motor bracket_v8 (Autodesk Fusion 360 design; units mm, degrees)
Autodesk Fusion 360 part; units mm, degrees
sketch "Sketch1" plane through (0, 0, 0) normal (0, 1, 0) x (1, 0, 0) in component "Component"
  line L0 (0, 0) -> (30.5, 0)
  line L1 (0, 0) -> (0, -30.5)
  line L2 (30.5, 0) -> (30.5, -3.5)
  line L3 (0, -30.5) -> (3.5, -30.5)
  line L4 (3.5, -30.5) -> (3.5, -3.5)
  line L5 (3.5, -3.5) -> (30.5, -3.5)
  dimension "d3" = 3.5
  dimension "d4" = 3.5
  dimension "d24" = 27
  dimension "d25" = 27
  constraint coincident L0.start L1.start
  constraint horizontal L0
  constraint perpendicular L0 L1
  constraint perpendicular L0 L2
  constraint perpendicular L1 L3
  constraint perpendicular L3 L4
  constraint perpendicular L2 L5
  measures "d3" distance of L0.end L2.end
  measures "d4" distance of L1.end L3.end
  measures "d24" distance of L3.end L4.end
  measures "d25" distance of L2.end L4.end
extrude "Extrude1" add sketch "Sketch1" along normal blind 38 in component "Component"
sketch "Sketch2" plane through (3.5, 0, 0) normal (1, 0, 0) x (0, 1, 0) in component "Component"
  line L0 (0, 30.5) -> (0, 3.5)
  line L1 (0, 3.5) -> (38, 3.5)
  line L2 (38, 3.5) -> (38, 30.5)
  line L3 (38, 30.5) -> (0, 30.5)
sketch "Sketch3" plane through (0, 0, 3.5) normal (0, 0, 1) x (-1, 0, 0) in component "Component"
  line L0 (-3.5, 0) -> (-30.5, 0)
  line L1 (-30.5, 0) -> (-30.5, -38)
  line L2 (-3.5, 0) -> (-3.5, -38) construction
  line L3 (-3.5, -19) -> (-10.25, -19) construction
  line L4 (-3.5, -38) -> (-3.5, 0) construction
  line L5 (0, 0) -> (0, -38) construction
  line L6 (-10.25, -19) -> (-10.25, -28) construction
  line L7 (-10.25, -28) -> (-23.75, -28) construction
  line L8 (-10.25, -28) -> (-10.25, -32) construction
  line L9 (-10.25, -32) -> (-8.5, -32) construction
  line L10 (-10.25, -28) -> (-8.5, -28) construction
  arc A0 (-12, -32) -> (-8.5, -32) centre (-10.25, -32) ccw
  arc A1 (-8.5, -28) -> (-12, -28) centre (-10.25, -28) ccw
  line L11 (-8.5, -28) -> (-8.5, -32)
  line L12 (-12, -28) -> (-12, -32)
  line L13 (-22, -28) -> (-22, -32)
  arc A2 (-22, -28) -> (-25.5, -28) centre (-23.75, -28) ccw
  line L14 (-25.5, -28) -> (-25.5, -32)
  arc A3 (-25.5, -32) -> (-22, -32) centre (-23.75, -32) ccw
  line L15 (-8.5, -10) -> (-8.5, -6)
  arc A4 (-12, -10) -> (-8.5, -10) centre (-10.25, -10) ccw
  line L16 (-12, -10) -> (-12, -6)
  arc A5 (-8.5, -6) -> (-12, -6) centre (-10.25, -6) ccw
  line L17 (-22, -10) -> (-22, -6)
  arc A6 (-25.5, -10) -> (-22, -10) centre (-23.75, -10) ccw
  line L18 (-25.5, -10) -> (-25.5, -6)
  arc A7 (-22, -6) -> (-25.5, -6) centre (-23.75, -6) ccw
  dimension "d27" = 6.75
  dimension "d28" = 9
  dimension "d29" = 13.5
  dimension "d30" = 4
  dimension "d31" = 1.75
  dimension "d34" = -13.5
  dimension "d35" = 0
  constraint coincident L0.start L2.start
  constraint perpendicular L0 L2
  constraint midpoint L2 L3.start
  constraint perpendicular L3 L4
  constraint equal L2 L5
  constraint perpendicular L3 L6
  constraint perpendicular L6 L7
  constraint perpendicular L7 L8
  constraint perpendicular L8 L9
  constraint perpendicular L8 L10
  constraint equal L9 L10
  constraint coincident L8.end L9.start
  constraint coincident L6.end L7.start
  constraint tangent A0 L12
  constraint tangent A1 L12
  constraint symmetric L3 L9.end L15.end
  constraint symmetric L3 L10.end L15.start
  constraint symmetric L3 A0.start L16.end
  constraint symmetric L3 A0 A5
  constraint symmetric L3 A1.end A4.start
  constraint symmetric L3 A1 A4
  constraint symmetric L3 L13.start L17.start
  constraint symmetric L3 L13.end L17.end
  constraint symmetric L3 A2.end A6.start
  constraint symmetric L3 A2 A6
  constraint symmetric L3 L14.end L18.end
  constraint symmetric L3 A3 A7
  measures "d27" distance of L3.start L3.end
  measures "d28" distance of L3.end L6.end
  measures "d29" distance of L6.end L7.end
  measures "d30" distance of L6.end L8.end
  measures "d31" distance of L8.end L9.end
extrude "Extrude3" cut sketch "Sketch3" against normal through all in component "Component"
sketch "Sketch2 (2)" plane through (3.5, 0, 0) normal (1, 0, 0) x (0, 1, 0)
  line L0 (0, 30.5) -> (0, 3.5) construction
  line L1 (0, 3.5) -> (38, 3.5) construction
  line L2 (38, 3.5) -> (38, 30.5) construction
  line L3 (38, 30.5) -> (0, 30.5) construction
  line L4 (19, 3.5) -> (19, 15) construction
  circle A0 centre (19, 15) radius 6.5
  line L5 (19, 15) -> (19, 22) construction
  line L6 (19, 22) -> (3.5, 22) construction
  circle A1 centre (3.5, 22) radius 1.75
  line L7 (19, 22) -> (11.25, 8.5766) construction
  circle A2 centre (11.25, 8.5766) radius 1.75
  circle A3 centre (34.5, 22) radius 1.75
  circle A4 centre (26.75, 8.5766) radius 1.75
  dimension "d37" = 11.5
  dimension "d38" = 13
  dimension "d39" = 7
  dimension "d40" = 15.5
  dimension "d41" = 3.5
  dimension "d42" = 60
  dimension "d43" = 3.5
  constraint midpoint L1 L4.start
  constraint perpendicular L1 L4
  constraint coincident L4.end A0.centre
  constraint parallel L4 L5
  constraint perpendicular L5 L6
  constraint coincident L6.end A1.centre
  constraint equal L6 L7
  constraint coincident L7.end A2.centre
  constraint symmetric L4 A1 A3
  constraint symmetric L4 A2 A4
  measures "d37" distance of L4.start L4.end
  measures "d38" diameter of A0
  measures "d39" distance of L4.end L5.end
  measures "d40" distance of L5.end L6.end
  measures "d41" diameter of A1
  measures "d42" angle of L6 L7
  measures "d43" diameter of A2
extrude "Extrude4" cut sketch "Sketch2 (2)" against normal through all in component "Component"
component "Component" placed x (1, 0, 0) y (0, 1, 0) z (0, 0, 1) at (0, 0, 0)
equation "d25 = d24"
equation "d28 = ( 18 / 2 ) * 1 mm"
equation "d31 = ( 3.5 / 2 ) * 1 mm"
equation "d40 = ( 31 / 2 ) * 1 mm"
equation "d42 = ( 360 / 6 ) * 1 deg"
equation "d43 = d41"
